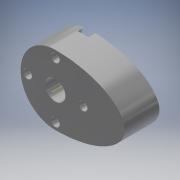
# Autodesk Inventor part: Дисковый кулачок
Saved by Autodesk Inventor 2019 (Build 230136000, 136)
## iProperties
Created: 2019-08-25
Part Number: Дисковый кулачок
Material: Stainless Steel, Austenitic
Document SubType Name: Modeling
Designer: Петров Иван
Manufacturer: Standard
Standards Organization: Custom
Density: 1 g/cm^3
Appearance: Steel
CustomPartVersion: 1
Author: Петров Иван
Autodesk Inventor part; units mm, degrees
ref_plane "YZ Plane" through (0, 0, 0) normal (1, 0, 0) x (0, 1, 0)
ref_plane "XZ Plane" through (0, 0, 0) normal (0, 1, 0) x (-1, 0, 0)
ref_plane "XY Plane" through (0, 0, 0) normal (0, 0, 1) x (1, 0, 0)
sketch "Основной эскиз" plane through (0, 0, 0) normal (0, 0, 1) x (1, 0, 0)
  spline S0 degree 5 poles (0, 10) (0.4903, 10.0023) (1.5101, 9.9783) (3.7169, 9.8863) (5.2913, 9.6625) (8.0626, 9.2068) (10.1701, 8.6378) (12.2795, 7.918) (14.0718, 7.1052) (15.6055, 6.2325) (16.8611, 5.3335) (17.8612, 4.439) (18.6277, 3.5746) (19.1912, 2.7582) (19.584, 1.9987) (19.8373, 1.2947) (19.9774, 0.635) (20.0219, 0) (19.9774, -0.635) (19.8373, -1.2947) (19.584, -1.9987) (19.1912, -2.7582) (18.6277, -3.5746) (17.8613, -4.439) (16.8611, -5.3335) (15.6056, -6.2325) (14.0715, -7.1052) (12.2803, -7.918) (10.1679, -8.6377) (8.0096, -9.223) (5.3353, -9.6504) (3.5804, -9.9121) (0.1193, -10.023) (-0.6801, -10.0105) (-2.0206, -9.8336) (-3.0596, -9.5465) (-4.0845, -9.1604) (-5.0112, -8.6841) (-5.8951, -8.1124) (-6.7092, -7.4519) (-7.4521, -6.7097) (-8.1123, -5.894) (-8.6841, -5.0137) (-9.1605, -4.0785) (-9.5367, -3.0987) (-9.8083, -2.0848) (-9.9725, -1.0482) (-10.0275, 0) (-9.9725, 1.0482) (-9.8083, 2.0848) (-9.5367, 3.0987) (-9.1605, 4.0785) (-8.6841, 5.0137) (-8.1122, 5.894) (-7.4522, 6.7097) (-6.7088, 7.4519) (-5.8961, 8.1123) (-5.0089, 8.6841) (-4.0898, 9.1603) (-3.1132, 9.5222) (-2.1817, 9.7972) (-1.2086, 9.9363) (-0.7293, 9.9855) (-0.3038, 9.9986) (0, 10) knots 0 0 0 0 0 0 0.029305 0.048463 0.072014 0.094795 0.11662 0.137346 0.156878 0.175161 0.192184 0.207975 0.22261 0.236216 0.248977 0.261135 0.272978 0.28482 0.296978 0.309739 0.323345 0.33798 0.353771 0.370794 0.389078 0.408609 0.429336 0.45116 0.473941 0.497492 0.519678 0.540296 0.559184 0.576225 0.59136 0.606495 0.621629 0.636764 0.651899 0.667034 0.682169 0.697304 0.712438 0.727573 0.742708 0.757843 0.772978 0.788112 0.803247 0.818382 0.833517 0.848652 0.863787 0.878921 0.894056 0.909191 0.924326 0.939461 0.954596 0.96973 0.981838 1 1 1 1 1 1
  point P0 (5.4767, 9.6166)
  point P1 (8.0209, 9.1553)
  point P2 (10.3525, 8.5413)
  point P3 (12.4298, 7.8038)
  point P4 (14.229, 6.9759)
  point P5 (15.7425, 6.0929)
  point P6 (16.977, 5.1896)
  point P7 (17.9502, 4.2975)
  point P8 (18.6889, 3.4429)
  point P9 (19.2256, 2.6435)
  point P10 (19.5949, 1.9073)
  point P11 (19.8303, 1.2315)
  point P12 (19.9592, 0.6029)
  point P13 (20, 0)
  point P14 (19.9592, -0.6029)
  point P15 (19.8303, -1.2315)
  point P16 (19.5949, -1.9073)
  point P17 (19.2256, -2.6435)
  point P18 (18.6889, -3.4429)
  point P19 (17.9502, -4.2975)
  point P20 (16.977, -5.1896)
  point P21 (15.7425, -6.0929)
  point P22 (14.229, -6.9759)
  point P23 (12.4298, -7.8038)
  point P24 (10.3525, -8.5413)
  point P25 (8.0209, -9.1553)
  point P26 (5.4767, -9.6166)
  point P27 (2.7788, -9.9029)
  point P28 (0, -10)
  point P29 (-1.0453, -9.9452)
  point P30 (-2.0791, -9.7815)
  point P31 (-3.0902, -9.5106)
  point P32 (-4.0674, -9.1355)
  point P33 (-5, -8.6603)
  point P34 (-5.8779, -8.0902)
  point P35 (-6.6913, -7.4314)
  point P36 (-7.4314, -6.6913)
  point P37 (-8.0902, -5.8779)
  point P38 (-8.6603, -5)
  point P39 (-9.1355, -4.0674)
  point P40 (-9.5106, -3.0902)
  point P41 (-9.7815, -2.0791)
  point P42 (-9.9452, -1.0453)
  point P43 (-10, 0)
  point P44 (-9.9452, 1.0453)
  point P45 (-9.7815, 2.0791)
  point P46 (-9.5106, 3.0902)
  point P47 (-9.1355, 4.0674)
  point P48 (-8.6603, 5)
  point P49 (-8.0902, 5.8779)
  point P50 (-7.4314, 6.6913)
  point P51 (-6.6913, 7.4314)
  point P52 (-5.8779, 8.0902)
  point P53 (-5, 8.6603)
  point P54 (-4.0674, 9.1355)
  point P55 (-3.0902, 9.5106)
  point P56 (-2.0791, 9.7815)
  point P57 (-1.0453, 9.9452)
  constraints: 60 other
extrude "Кулачок" add sketch "Основной эскиз" along normal blind 10
sketch "Эскиз2" plane through (0, 0, 10) normal (0, 0, 1) x (1, 0, 0)
  arc A0 (-0.25, 9.2247) -> (0.25, 9.2247) centre (0, 8) ccw
  line L0 (-0.25, 10.9972) -> (-0.25, 9.2247)
  arc A1 (-0.25, 10.9972) -> (-1.1469, -10.94) centre (0, 0) ccw
  line L1 (-1.1469, -10.6297) -> (-1.1469, -10.94)
  line L2 (-0.8473, -10.6297) -> (-1.1469, -10.6297)
  line L3 (-0.8473, -10.9673) -> (-0.8473, -10.6297)
  arc A2 (-0.8473, -10.9673) -> (0.8535, -10.9668) centre (0, 0) ccw
  line L4 (0.8535, -10.6297) -> (0.8535, -10.9668)
  line L5 (1.1541, -10.6297) -> (0.8535, -10.6297)
  line L6 (1.1541, -10.9393) -> (1.1541, -10.6297)
  arc A3 (1.1541, -10.9393) -> (0.25, 10.9972) centre (0, 0) ccw
  line L7 (0.25, 9.2247) -> (0.25, 10.9972)
  circle A4 centre (8, 0) radius 1.25
  circle A5 centre (0, -8) radius 1.25
  circle A6 centre (-8, 0) radius 1.25
  circle A7 centre (0, -5.5) radius 0.75
  circle A8 centre (4.7631, 2.75) radius 0.75
  circle A9 centre (-4.7631, 2.75) radius 0.75
  circle A10 centre (0, 0) radius 2.9
  arc A11 (0.25, 9.2247) -> (-0.25, 9.2247) centre (0, 8) ccw
  constraints: 16 end point, 12 centre point, 10 point on circle
extrude "Выдавливание2" cut sketch "Эскиз2" against normal blind 10 contours A11 A0 | A4 | A5 | A6
sketch "Эскиз3" plane through (0, 0, 10) normal (0, 0, 1) x (1, 0, 0)
  arc A0 (-0.25, 9.2247) -> (0.25, 9.2247) centre (0, 8) ccw
  line L0 (-0.25, 10.9972) -> (-0.25, 9.2247)
  arc A1 (-0.25, 10.9972) -> (-1.1469, -10.94) centre (0, 0) ccw
  line L1 (-1.1469, -10.6297) -> (-1.1469, -10.94)
  line L2 (-0.8473, -10.6297) -> (-1.1469, -10.6297)
  line L3 (-0.8473, -10.9673) -> (-0.8473, -10.6297)
  arc A2 (-0.8473, -10.9673) -> (0.8535, -10.9668) centre (0, 0) ccw
  line L4 (0.8535, -10.6297) -> (0.8535, -10.9668)
  line L5 (1.1541, -10.6297) -> (0.8535, -10.6297)
  line L6 (1.1541, -10.9393) -> (1.1541, -10.6297)
  arc A3 (1.1541, -10.9393) -> (0.25, 10.9972) centre (0, 0) ccw
  line L7 (0.25, 9.2247) -> (0.25, 10.9972)
  circle A4 centre (8, 0) radius 1.25
  circle A5 centre (0, -8) radius 1.25
  circle A6 centre (-8, 0) radius 1.25
  circle A7 centre (0, -5.5) radius 0.75
  circle A8 centre (4.7631, 2.75) radius 0.75
  circle A9 centre (-4.7631, 2.75) radius 0.75
  circle A10 centre (0, 0) radius 2.9
  arc A11 (0.25, 9.2247) -> (-0.25, 9.2247) centre (0, 8) ccw
  constraints: 16 end point, 12 centre point, 10 point on circle
extrude "Выдавливание3" cut sketch "Эскиз3" against normal blind 7 contours A10
sketch "Эскиз4" plane through (0, 0, 0) normal (0, 0, -1) x (-1, 0, 0)
  circle A0 centre (0, 0) radius 2
  dimension "d8" = 4
  constraints: 1 centre point, 1 coincident
  measures "d8" diameter of A0
extrude "Выдавливание4" cut sketch "Эскиз4" against normal blind 7
sketch "Эскиз5" plane through (0, 0, 0) normal (0, 0, -1) x (-1, 0, 0)
  circle A0 centre (0, 8) radius 1.25 projected
  circle A1 centre (0, 8) radius 2.5
  circle A2 centre (8, 0) radius 1.25 projected
  circle A3 centre (8, 0) radius 2.5
  circle A4 centre (0, -8) radius 1.25 projected
  circle A5 centre (0, -8) radius 2.5
  circle A6 centre (-8, 0) radius 1.25 projected
  circle A7 centre (-8, 0) radius 2.5
  point P0 (0, 0)
  dimension "d11" = 5
  dimension "d12" = 5
  dimension "d13" = 5
  dimension "d14" = 5
  constraints: 4 centre point, 4 coincident
  measures "d11" diameter of A1
  measures "d12" diameter of A3
  measures "d13" diameter of A5
  measures "d14" diameter of A7
extrude "Выдавливание5" cut sketch "Эскиз5" against normal blind 2 contours A0 | A1 | A2 | A3 | A4 | A5 | A6 | A7
body "Solid1"
